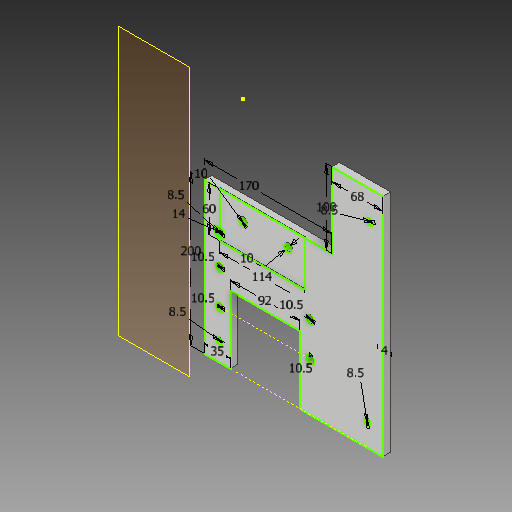
# Autodesk Inventor part: Part1
Saved by Autodesk Inventor 2018 (Build 220112000, 112)
## iProperties
Created: 2017-06-06
Part Number: Part1
Material: Generic
Document SubType Name: Modeling
Designer: m228540
Density: 1 g/cm^3
Appearance: Default
Author: m228540
Autodesk Inventor part; units mm, degrees
ref_plane "YZ Plane" through (0, 0, 0) normal (1, 0, 0) x (0, 1, 0)
ref_plane "XZ Plane" through (0, 0, 0) normal (0, 1, 0) x (-1, 0, 0)
ref_plane "XY Plane" through (0, 0, 0) normal (0, 0, 1) x (1, 0, 0)
ref_plane "Work Plane1" through (678.6266, 4, 0) normal (0, 0, 1) x (1, 0, 0)
sketch "Sketch1" plane through (678.6266, 4, 0) normal (0, 0, 1) x (1, 0, 0)
  circle A0 centre (-710.3818, -172.4297) radius 4.25
  line L0 (-690.3818, -322.4297) -> (-513.3818, -322.4297) construction
  circle A1 centre (-679.3818, -145.4297) radius 5
  circle A2 centre (-619.3818, -145.4297) radius 5
  line L1 (-730.3818, -322.4297) -> (-695.3818, -322.4297)
  line L2 (-695.3818, -322.4297) -> (-695.3818, -232.4297)
  line L3 (-695.3818, -232.4297) -> (-603.3818, -232.4297)
  line L4 (-603.3818, -232.4297) -> (-603.3818, -322.4297)
  circle A3 centre (-710.3818, -172.4297) radius 4.25
  circle A4 centre (-513.3818, -292.4297) radius 4.25
  circle A5 centre (-510.3818, -60.4297) radius 4.25
  line L5 (-488.3818, -194.7007) -> (-492.3818, -194.7007)
  line L6 (-492.3818, -194.7007) -> (-492.3818, -322.4297)
  line L7 (-492.3818, -322.4297) -> (-492.3818, -22.4297)
  line L8 (-492.3818, -322.4297) -> (-603.3818, -322.4297)
  line L9 (-555.3818, -22.4297) -> (-492.3818, -22.4297)
  line L10 (-492.3818, -22.4297) -> (-560.3818, -22.4297)
  line L11 (-560.3818, -22.4297) -> (-560.3818, -120.4297)
  circle A6 centre (-710.3818, -297.4297) radius 4.25
  line L12 (-560.3818, -22.4297) -> (-560.3818, -122.4297)
  line L13 (-560.3818, -122.4297) -> (-730.3818, -122.4297)
  line L14 (-730.3818, -322.4297) -> (-730.3818, -122.4297)
  line L15 (-710.3818, -122.4297) -> (-710.3818, -182.4297)
  line L16 (-710.3818, -182.4297) -> (-596.3818, -182.4297)
  line L17 (-596.3818, -182.4297) -> (-596.3818, -122.4297)
  circle A7 centre (-710.3818, -172.4297) radius 7
  circle A8 centre (-709.3818, -258.4297) radius 5.25
  circle A9 centre (-709.3818, -212.4297) radius 5.25
  line L18 (-709.3818, -258.4297) -> (-589.3818, -258.4297) construction
  circle A10 centre (-589.3818, -258.4297) radius 5.25
  circle A11 centre (-589.3818, -212.4297) radius 5.25
  point P0 (-678.6266, -4)
  dimension "d52" = 8.5
  dimension "d57" = 10
  dimension "d59" = 10
  dimension "d61" = 35
  dimension "d62" = 92
  dimension "d70" = 8.5
  dimension "d71" = 8.5
  dimension "d72" = 4
  dimension "d73" = 68
  dimension "d75" = 8.5
  dimension "d76" = 100
  dimension "d77" = 200
  dimension "d78" = 170
  dimension "d80" = 60
  dimension "d81" = 114
  dimension "d88" = 14
  dimension "d95" = 10.5
  dimension "d96" = 10.5
  dimension "d100" = 10.5
  dimension "d101" = 10.5
  constraints: 38 end point, 12 centre point, 5 perpendicular, 5 point on line, 3 coincident, 2 horizontal, 1 concentric, 1 vertical
  measures "d52" diameter of A0
  measures "d57" diameter of A1
  measures "d59" diameter of A2
  measures "d61" distance of L1.start L1.end
  measures "d62" distance of L2.end L3.end
  measures "d70" diameter of A4
  measures "d71" diameter of A5
  measures "d72" distance of L5.start L5.end
  measures "d73" distance of L7.end L10.end
  measures "d75" diameter of A6
  measures "d76" distance of L10.end L12.end
  measures "d77" distance of L1.start L13.end
  measures "d78" distance of L12.end L13.end
  measures "d80" distance of L15.start L15.end
  measures "d81" distance of L15.end L16.end
  measures "d88" diameter of A7
  measures "d95" diameter of A8
  measures "d96" diameter of A9
  measures "d100" diameter of A10
  measures "d101" diameter of A11
extrude "Extrusion5" add sketch "Sketch1" against normal blind 10 contours A0 L15 | A0 L15 A7 | L15 A0 | A0 L15 A7 | A7 L15 L16 L17 L13 L12 L11 L10 L9 L7 L6 L8 L4 L3 L2 L1 L14 | L15 L13 L17 L16 A7 | A8 | A9 | A10 | A11
extrude "Extrusion7" cut sketch "Sketch1" against normal blind 1.5 contours A0 L15 | A0 L15 A7 | L15 L13 L17 L16 A7 picked at (-708.9651, -172.4297) picked at (-709.5473, -178.419)
extrude "Extrusion6" cut sketch "Sketch1" against normal blind 10 contours A0 L15 | L15 A0
extrude "Extrusion8" cut sketch "Sketch1" against normal blind 1.5 contours A0 L15 A7 | A0 L15 A7
extrude "Extrusion9" cut sketch "Sketch1" against normal blind 10.5 contours A8 | A9 | A10 | A11
body "Solid2"
